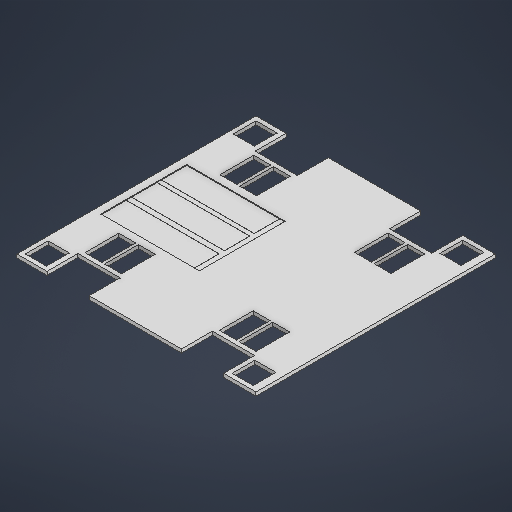
# Autodesk Inventor part: base
Saved by Autodesk Inventor 2026.2 (Build 302298010, 298A)
## iProperties
Created: 2026-03-12
Part Number: base
Material: Generic
Document SubType Name: Modeling
Designer: karol
Density: 1 g/cm^3
Appearance: Default
Author: karol
Autodesk Inventor part; units mm, degrees
ref_plane "YZ Plane" through (0, 0, 0) normal (1, 0, 0) x (0, 1, 0)
ref_plane "XZ Plane" through (0, 0, 0) normal (0, 1, 0) x (-1, 0, 0)
ref_plane "XY Plane" through (0, 0, 0) normal (0, 0, 1) x (1, 0, 0)
sketch "Sketch3" plane through (0, 0, 0) normal (0, 1, 0) x (-1, 0, 0)
  line L0 (0, 0) -> (170, 0)
  line L1 (170, 0) -> (170, -170)
  line L2 (170, -170) -> (0, -170)
  line L3 (0, -170) -> (0, 0)
  line L4 (170, 0) -> (167, 0)
  line L5 (167, 0) -> (167, -170)
  line L6 (167, -170) -> (170, -170)
  line L7 (170, -170) -> (170, 0)
  line L8 (167, 0) -> (148.6, 0)
  line L9 (148.6, 0) -> (148.6, -3)
  line L10 (148.6, -3) -> (167, -3)
  line L11 (167, -3) -> (167, 0)
  line L12 (148.6, -3) -> (151.6, -3)
  line L13 (151.6, -3) -> (151.6, -25)
  line L14 (151.6, -25) -> (148.6, -25)
  line L15 (148.6, -25) -> (148.6, -3)
  line L16 (167, -170) -> (148.6, -170)
  line L17 (148.6, -170) -> (148.6, -167)
  line L18 (148.6, -167) -> (167, -167)
  line L19 (167, -167) -> (167, -170)
  line L20 (148.6, -167) -> (151.6, -167)
  line L21 (151.6, -167) -> (151.6, -145)
  line L22 (151.6, -145) -> (148.6, -145)
  line L23 (148.6, -145) -> (148.6, -167)
  line L24 (167, -167) -> (152, -167)
  line L25 (152, -167) -> (152, -150.8)
  line L26 (152, -150.8) -> (167, -150.8)
  line L27 (167, -150.8) -> (167, -167)
  line L28 (167, -3) -> (152, -3)
  line L29 (152, -3) -> (152, -19.2)
  line L30 (152, -19.2) -> (167, -19.2)
  line L31 (167, -19.2) -> (167, -3)
  line L32 (148.6, -25) -> (118.6, -25)
  line L33 (118.6, -25) -> (118.6, 0)
  line L34 (118.6, 0) -> (148.6, 0)
  line L35 (148.6, 0) -> (148.6, -25)
  line L36 (148.6, -145) -> (118.6, -145)
  line L37 (118.6, -145) -> (118.6, -170)
  line L38 (118.6, -170) -> (148.6, -170)
  line L39 (148.6, -170) -> (148.6, -145)
  line L40 (0, 0) -> (20, 0)
  line L41 (20, 0) -> (20, -3)
  line L42 (20, -3) -> (0, -3)
  line L43 (0, -3) -> (0, 0)
  line L44 (0, -170) -> (20, -170)
  line L45 (20, -170) -> (20, -167)
  line L46 (20, -167) -> (0, -167)
  line L47 (0, -167) -> (0, -170)
  line L48 (20, -3) -> (5, -3)
  line L49 (5, -3) -> (5, -19.2)
  line L50 (5, -19.2) -> (20, -19.2)
  line L51 (20, -19.2) -> (20, -3)
  line L52 (20, -167) -> (5, -167)
  line L53 (5, -167) -> (5, -150.8)
  line L54 (5, -150.8) -> (20, -150.8)
  line L55 (20, -150.8) -> (20, -167)
  line L56 (20, 0) -> (23, 0)
  line L57 (23, 0) -> (23, -25)
  line L58 (23, -25) -> (20, -25)
  line L59 (20, -25) -> (20, 0)
  line L60 (23, -25) -> (53, -25)
  line L61 (53, -25) -> (53, 0)
  line L62 (53, 0) -> (23, 0)
  line L63 (23, 0) -> (23, -25)
  line L64 (53, 0) -> (56, 0)
  line L65 (56, 0) -> (56, -25)
  line L66 (56, -25) -> (53, -25)
  line L67 (53, -25) -> (53, 0)
  line L68 (53, -25) -> (23, -25)
  line L69 (23, -25) -> (23, -22)
  line L70 (23, -22) -> (53, -22)
  line L71 (53, -22) -> (53, -25)
  line L72 (148.6, -25) -> (118.6, -25)
  line L73 (118.6, -25) -> (118.6, -22)
  line L74 (118.6, -22) -> (148.6, -22)
  line L75 (148.6, -22) -> (148.6, -25)
  line L76 (118.6, -25) -> (115.6, -25)
  line L77 (115.6, -25) -> (115.6, 0)
  line L78 (115.6, 0) -> (118.6, 0)
  line L79 (118.6, 0) -> (118.6, -25)
  line L80 (148.6, -145) -> (118.6, -145)
  line L81 (118.6, -145) -> (118.6, -148)
  line L82 (118.6, -148) -> (148.6, -148)
  line L83 (148.6, -148) -> (148.6, -145)
  line L84 (118.6, -145) -> (115.6, -145)
  line L85 (115.6, -145) -> (115.6, -170)
  line L86 (115.6, -170) -> (118.6, -170)
  line L87 (118.6, -170) -> (118.6, -145)
  line L88 (20, -170) -> (23, -170)
  line L89 (23, -170) -> (23, -145)
  line L90 (23, -145) -> (20, -145)
  line L91 (20, -145) -> (20, -170)
  line L92 (23, -170) -> (53, -170)
  line L93 (53, -170) -> (53, -145)
  line L94 (53, -145) -> (23, -145)
  line L95 (23, -145) -> (23, -170)
  line L96 (53, -145) -> (56, -145)
  line L97 (56, -145) -> (56, -170)
  line L98 (56, -170) -> (53, -170)
  line L99 (53, -170) -> (53, -145)
  line L100 (53, -145) -> (23, -145)
  line L101 (23, -145) -> (23, -148)
  line L102 (23, -148) -> (53, -148)
  line L103 (53, -148) -> (53, -145)
  line L104 (148.6, -25) -> (146.6, -25)
  line L105 (146.6, -25) -> (146.6, -49)
  line L106 (146.6, -49) -> (148.6, -49)
  line L107 (148.6, -49) -> (148.6, -25)
  line L108 (118.6, -25) -> (120.6, -25)
  line L109 (120.6, -25) -> (120.6, -49)
  line L110 (120.6, -49) -> (118.6, -49)
  line L111 (118.6, -49) -> (118.6, -25)
  line L112 (146.6, -25) -> (134.6, -25)
  line L113 (134.6, -25) -> (134.6, -49)
  line L114 (134.6, -49) -> (146.6, -49)
  line L115 (146.6, -49) -> (146.6, -25)
  line L116 (120.6, -49) -> (132.6, -49)
  line L117 (132.6, -49) -> (132.6, -25)
  line L118 (132.6, -25) -> (120.6, -25)
  line L119 (120.6, -25) -> (120.6, -49)
  line L120 (148.6, -145) -> (146.6, -145)
  line L121 (146.6, -145) -> (146.6, -121)
  line L122 (146.6, -121) -> (148.6, -121)
  line L123 (148.6, -121) -> (148.6, -145)
  line L124 (118.6, -145) -> (120.6, -145)
  line L125 (120.6, -145) -> (120.6, -121)
  line L126 (120.6, -121) -> (118.6, -121)
  line L127 (118.6, -121) -> (118.6, -145)
  line L128 (146.6, -121) -> (134.6, -121)
  line L129 (134.6, -121) -> (134.6, -145)
  line L130 (134.6, -145) -> (146.6, -145)
  line L131 (146.6, -145) -> (146.6, -121)
  line L132 (120.6, -121) -> (132.6, -121)
  line L133 (132.6, -121) -> (132.6, -145)
  line L134 (132.6, -145) -> (120.6, -145)
  line L135 (120.6, -145) -> (120.6, -121)
  line L136 (53, -25) -> (51, -25)
  line L137 (51, -25) -> (51, -60.37)
  line L138 (51, -60.37) -> (53, -60.37)
  line L139 (53, -60.37) -> (53, -25)
  line L140 (51, -25) -> (39, -25)
  line L141 (39, -25) -> (39, -60.37)
  line L142 (39, -60.37) -> (51, -60.37)
  line L143 (51, -60.37) -> (51, -25)
  line L144 (23, -25) -> (25, -25)
  line L145 (25, -25) -> (25, -60.37)
  line L146 (25, -60.37) -> (23, -60.37)
  line L147 (23, -60.37) -> (23, -25)
  line L148 (25, -25) -> (37, -25)
  line L149 (37, -25) -> (37, -60.37)
  line L150 (37, -60.37) -> (25, -60.37)
  line L151 (25, -60.37) -> (25, -25)
  line L152 (53, -145) -> (51, -145)
  line L153 (51, -145) -> (51, -121)
  line L154 (51, -121) -> (53, -121)
  line L155 (53, -121) -> (53, -145)
  line L156 (51, -121) -> (39, -121)
  line L157 (39, -121) -> (39, -145)
  line L158 (39, -145) -> (51, -145)
  line L159 (51, -145) -> (51, -121)
  line L160 (23, -145) -> (25, -145)
  line L161 (25, -145) -> (25, -121)
  line L162 (25, -121) -> (23, -121)
  line L163 (23, -121) -> (23, -145)
  line L164 (25, -121) -> (37, -121)
  line L165 (37, -121) -> (37, -145)
  line L166 (37, -145) -> (25, -145)
  line L167 (25, -145) -> (25, -121)
  line L168 (118.6, -25) -> (115.6, -25)
  line L169 (115.6, -25) -> (115.6, 0)
  line L170 (115.6, 0) -> (118.6, 0)
  line L171 (118.6, 0) -> (118.6, -25)
  line L172 (115.6, 0) -> (56, 0)
  line L173 (56, 0) -> (56, -3)
  line L174 (56, -3) -> (115.6, -3)
  line L175 (115.6, -3) -> (115.6, 0)
  line L176 (115.6, -170) -> (56, -170)
  line L177 (56, -170) -> (56, -167)
  line L178 (56, -167) -> (115.6, -167)
  line L179 (115.6, -167) -> (115.6, -170)
  line L180 (51, -25) -> (39, -25)
  line L181 (39, -25) -> (39, -49)
  line L182 (39, -49) -> (51, -49)
  line L183 (51, -49) -> (51, -25)
  line L184 (37, -25) -> (25, -25)
  line L185 (25, -25) -> (25, -49)
  line L186 (25, -49) -> (37, -49)
  line L187 (37, -49) -> (37, -25)
  dimension "d108" = 170
  dimension "d109" = 170
  dimension "d110" = 3
  dimension "d111" = 18.4
  dimension "d112" = 3
  dimension "d113" = 22
  dimension "d114" = 3
  dimension "d115" = 3
  dimension "d116" = 22
  dimension "d117" = 3
  dimension "d118" = 15
  dimension "d119" = 16.2
  dimension "d120" = 15
  dimension "d121" = 16.2
  dimension "d122" = 30
  dimension "d123" = 30
  dimension "d124" = 20
  dimension "d125" = 15
  dimension "d126" = 3
  dimension "d127" = 25
  dimension "d128" = 25
  dimension "d129" = 30
  dimension "d130" = 3
  dimension "d131" = 3
  dimension "d132" = 3
  dimension "d133" = 3
  dimension "d134" = 3
  dimension "d135" = 2
  dimension "d136" = 24
  dimension "d137" = 2
  dimension "d138" = 24
  dimension "d139" = 12
  dimension "d140" = 12
  dimension "d141" = 24
  dimension "d142" = 2
  dimension "d143" = 12
  dimension "d144" = 2
  dimension "d145" = 12
  dimension "d146" = 3
  dimension "d147" = 3
  dimension "d150" = 24
  dimension "d151" = 35.37
  dimension "d152" = 24
  dimension "d153" = 24
  dimension "d154" = 24
  dimension "d155" = 24
  constraints: 376 end point, 94 parallel, 47 horizontal, 47 perpendicular, 32 point on line
  measures "d108" distance of L1.end L2.end
  measures "d109" distance of L0.end L1.end
  measures "d110" distance of L6.end L5.end
  measures "d111" distance of L10.end L9.end
  measures "d112" distance of L13.end L14.end
  measures "d113" distance of L12.end L13.end
  measures "d114" distance of L8.end L9.end
  measures "d115" distance of L16.end L17.end
  measures "d116" distance of L21.end L20.end
  measures "d117" distance of L21.end L22.end
  measures "d118" distance of L25.end L26.end
  measures "d119" distance of L24.end L25.end
  measures "d120" distance of L30.end L29.end
  measures "d121" distance of L29.end L28.end
  measures "d122" distance of L33.end L34.end
  measures "d123" distance of L38.end L37.end
  measures "d124" distance of L41.end L42.end
  measures "d125" distance of L50.end L49.end
  measures "d126" distance of L57.end L58.end
  measures "d127" distance of L32.end L33.end
  measures "d128" distance of L56.end L57.end
  measures "d129" distance of L62.end L61.end
  measures "d130" distance of L65.end L66.end
  measures "d131" distance of L68.end L69.end
  measures "d132" distance of L77.end L78.end
  measures "d133" distance of L81.end L80.end
  measures "d134" distance of L86.end L85.end
  measures "d135" distance of L106.end L105.end
  measures "d136" distance of L105.end L104.end
  measures "d137" distance of L109.end L110.end
  measures "d138" distance of L108.end L109.end
  measures "d139" distance of L114.end L113.end
  measures "d140" distance of L118.end L117.end
  measures "d141" distance of L120.end L121.end
  measures "d142" distance of L138.end L137.end
  measures "d143" distance of L142.end L141.end
  measures "d144" distance of L145.end L146.end
  measures "d145" distance of L149.end L150.end
  measures "d146" distance of L173.end L172.end
  measures "d147" distance of L176.end L177.end
  measures "d150" distance between parallel lines of L36 L132
  measures "d151" distance between parallel lines of L142 L140
  measures "d152" distance of L181.end L180.end
  measures "d153" distance of L185.end L184.end
  measures "d154" distance between parallel lines of L158 L156
  measures "d155" distance between parallel lines of L94 L164
extrude "Extrusion3" add sketch "Sketch3" along normal blind 2.5 contours L0 L41 L42 L3 | L0 L57 L58 L59 L51 L41 | L42 L49 L50 L59 L58 L147 L146 L150 L149 L60 L141 L142 L138 L139 L66 L65 L174 L77 L76 L111 L110 L116 L117 L32 L113 L114 L106 L107 L14 L13 L10 L29 L30 L5 L26 L25 L18 L21 L22 L123 L122 L128 L129 L36 L133 L132 L126 L127 L84 L85 L178 L97 L96 L155 L154 L156 L157 L94 L165 L164 L162 L163 L90 L91 L54 L53 L46 L3 | L46 L45 L2 L3 | L0 L65 L66 L61 | L70 L61 L60 L57 | L0 L77 L174 L65 | L60 L145 L146 L147 | L45 L55 L91 L90 L89 L2 | L0 L33 L76 L77 | L139 L138 L137 L60 | L186 L149 L150 L145 | L93 L96 L97 L2 | L89 L94 L93 L102 | L0 L5 L10 L9 | L74 L15 L32 L33 | L137 L142 L141 L182 | L97 L178 L85 L2 | L163 L162 L161 L94 | L0 L1 L2 L5 | L10 L13 L14 L15 | L32 L109 L110 L111 | L85 L84 L37 L2 | L94 L153 L154 L155 | L107 L106 L105 L32 | L17 L18 L5 L2 | L37 L36 L23 L82 | L23 L22 L21 L18 | L127 L126 L125 L36 | L36 L121 L122 L123
sketch "Sketch4" plane through (0, 2.5, 0) normal (0, 1, 0) x (1, 0, 0)
  line L0 (-134.6, 121) -> (-146.6, 121) projected
  line L1 (-132.6, 49) -> (-120.6, 49) projected
  line L2 (-146.6, 121) -> (-120.6, 121)
  line L3 (-120.6, 121) -> (-120.6, 49)
  line L4 (-120.6, 49) -> (-146.6, 49)
  line L5 (-146.6, 49) -> (-146.6, 121)
  line L6 (-146.6, 121) -> (-120.6, 121)
  line L7 (-120.6, 121) -> (-120.6, 115.5)
  line L8 (-120.6, 115.5) -> (-146.6, 115.5)
  line L9 (-146.6, 115.5) -> (-146.6, 121)
  line L10 (-146.6, 49) -> (-120.6, 49)
  line L11 (-120.6, 49) -> (-120.6, 54.5)
  line L12 (-120.6, 54.5) -> (-146.6, 54.5)
  line L13 (-146.6, 54.5) -> (-146.6, 49)
  line L14 (-164.7573, 115.5) -> (-94.7573, 115.5)
  line L15 (-94.7573, 115.5) -> (-94.7573, 54.5)
  line L16 (-94.7573, 54.5) -> (-164.7573, 54.5)
  line L17 (-164.7573, 54.5) -> (-164.7573, 115.5)
  point P0 (0, 0)
  dimension "d156" = 5.5
  dimension "d157" = 5.5
  dimension "d158" = 70
  constraints: 32 end point, 8 parallel, 4 horizontal, 4 perpendicular, 2 point on line
  measures "d156" distance of L6.end L7.end
  measures "d157" distance of L11.end L10.end
  measures "d158" distance of L15.end L16.end
extrude "Extrusion4" cut sketch "Sketch4" against normal blind 0.5 contours L8 L3 L12 L5 | L5 L16 L17 L14 | L14 L15 L16 L3
sketch "Sketch5" plane through (0, 2, 0) normal (0, 1, 0) x (1, 0, 0)
  line L0 (-164.7573, 54.5) -> (-164.7573, 115.5) projected
  line L1 (-164.7573, 115.5) -> (-98.7573, 115.5)
  line L2 (-98.7573, 115.5) -> (-98.7573, 97.5)
  line L3 (-98.7573, 97.5) -> (-164.7573, 97.5)
  line L4 (-164.7573, 97.5) -> (-164.7573, 115.5)
  line L5 (-164.7573, 54.5) -> (-98.7573, 54.5)
  line L6 (-98.7573, 54.5) -> (-98.7573, 72.5)
  line L7 (-98.7573, 72.5) -> (-164.7573, 72.5)
  line L8 (-164.7573, 72.5) -> (-164.7573, 54.5)
  line L9 (-164.7573, 94.324) -> (-98.7573, 94.324)
  line L10 (-98.7573, 94.324) -> (-98.7573, 76.324)
  line L11 (-98.7573, 76.324) -> (-164.7573, 76.324)
  line L12 (-164.7573, 76.324) -> (-164.7573, 94.324)
  point P0 (0, 0)
  dimension "d161" = 66
  dimension "d162" = 18
  dimension "d163" = 66
  dimension "d164" = 18
  dimension "d165" = 66
  dimension "d166" = 18
  constraints: 24 end point, 6 parallel, 3 horizontal, 3 perpendicular, 1 point on line
  measures "d161" distance of L2.end L3.end
  measures "d162" distance of L1.end L2.end
  measures "d163" distance of L7.end L6.end
  measures "d164" distance of L6.end L5.end
  measures "d165" distance of L10.end L11.end
  measures "d166" distance of L9.end L10.end
extrude "Extrusion5" cut sketch "Sketch5" against normal blind 0.1
body "Solid2"
